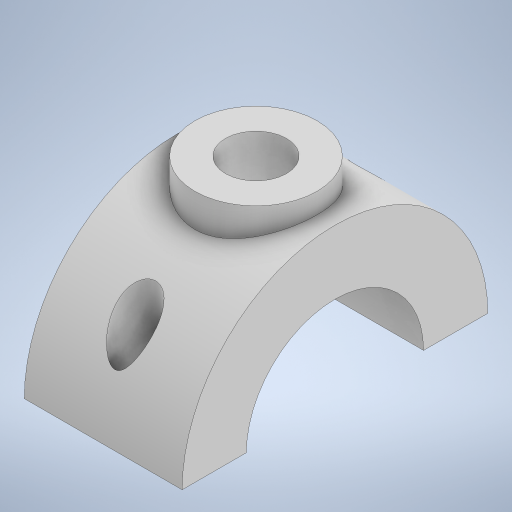
# Autodesk Inventor part: Parte1
Saved by Autodesk Inventor 2023 (Build 270158000, 158)
## iProperties
Created: 2022-11-03
Part Number: Parte1
Material: Generic
Document SubType Name: Modeling
Designer: ivanm
Density: 1 g/cm^3
Appearance: Default
Author: ivanm
Autodesk Inventor part; units mm, degrees
ref_plane "YZ Plane" through (0, 0, 0) normal (1, 0, 0) x (0, 1, 0)
ref_plane "XZ Plane" through (0, 0, 0) normal (0, 1, 0) x (-1, 0, 0)
ref_plane "XY Plane" through (0, 0, 0) normal (0, 0, 1) x (1, 0, 0)
sketch "Sketch1" plane through (0, 0, 0) normal (1, 0, 0) x (0, 1, 0)
  arc A0 (0, -8.7) -> (0, 8.7) centre (0, 0) ccw
  arc A1 (0, -15) -> (0, 15) centre (0, 0) ccw
  line L0 (0, 15) -> (0, 8.7)
  line L1 (0, -8.7) -> (0, -15)
  dimension "d0" = 17.4
  dimension "d1" = 30
  dimension "d17" = 6.3
  dimension "d18" = 6.3
  constraints: 4 end point, 4 point on circle, 3 coincident, 2 centre point, 2 vertical
  measures "d0" diameter of A0
  measures "d1" diameter of A1
  measures "d17" distance of L0.start L0.end
  measures "d18" distance of L1.start L1.end
extrude "Extrusion1" add sketch "Sketch1" along normal blind 15.5
ref_plane "Work Plane1" through (0, 15, 0) normal (0, -1, 0) x (1, 0, 0)
sketch "Sketch2" plane through (0, 15, 0) normal (0, -1, 0) x (1, 0, 0)
  line L0 (0, -15) -> (0, 15) projected
  line L1 (0, 15) -> (15.5, 15) projected
  line L2 (15.5, -15) -> (15.5, 15) projected
  line L3 (0, -15) -> (15.5, -15) projected
  line L4 (0, 0) -> (15.5, 0) construction
  line L5 (7.75, -15) -> (7.75, 15) construction
  circle A0 centre (7.75, 0) radius 6
  circle A1 centre (7.75, 0) radius 3
  dimension "d6" = 6
  dimension "d7" = 12
  constraints: 4 end point, 4 midpoint, 2 centre point, 1 coincident, 1 perpendicular
  measures "d6" diameter of A1
  measures "d7" diameter of A0
extrude "Extrusion2" add sketch "Sketch2" along normal up to surface contours A0 round surface about axis through (0, 0, 0) along (1, 0, 0) radius 15 far side no
extrude "Extrusion3" add sketch "Sketch2" against normal blind 2 contours A0
extrude "Extrusion4" cut sketch "Sketch2" along normal through all contours A1
ref_plane "Work Plane2" through (0, -8.7, 0) normal (0, -1, 0) x (1, 0, 0)
sketch "Sketch3" plane through (0, -8.7, 0) normal (0, -1, 0) x (1, 0, 0)
  spline S0 degree 5 poles (10.75, 0) (10.75, 0.1919) (10.7347, 0.3834) (10.7041, 0.5715) (10.6595, 0.7536) (10.4842, 1.2932) (10.3128, 1.6211) (10.104, 1.9046) (9.8731, 2.1435) (9.2912, 2.6088) (8.9274, 2.8036) (8.5449, 2.9327) (8.1539, 2.9984) (7.3698, 3.0016) (6.9775, 2.9389) (6.5935, 2.8124) (6.2279, 2.62) (5.7133, 2.2146) (5.5421, 2.0519) (5.3825, 1.8674) (5.238, 1.6607) (5.0376, 1.2915) (4.969, 1.1429) (4.9094, 0.9866) (4.86, 0.8234) (4.7677, 0.4105) (4.7372, 0.1545) (4.7351, -0.1058) (4.7615, -0.3627) (4.8805, -0.9375) (4.9927, -1.2467) (5.1399, -1.5242) (5.3101, -1.7688) (5.6294, -2.1312) (5.7684, -2.2647) (5.9146, -2.3841) (6.0665, -2.4898) (6.5084, -2.751) (6.8094, -2.8759) (7.1199, -2.9586) (7.4347, -3) (8.1471, -3) (8.5437, -2.9342) (8.9317, -2.8031) (9.3003, -2.6045) (9.8094, -2.1928) (9.9736, -2.0335) (10.127, -1.8538) (10.2662, -1.653) (10.5189, -1.1875) (10.6303, -0.9149) (10.7095, -0.6203) (10.75, -0.3119) (10.75, 0) knots 0 0 0 0 0 0 0.042105 0.042105 0.042105 0.042105 0.130974 0.130974 0.130974 0.130974 0.2493 0.2493 0.2493 0.2493 0.367924 0.367924 0.367924 0.367924 0.431887 0.431887 0.431887 0.431887 0.470966 0.470966 0.470966 0.470966 0.527372 0.527372 0.527372 0.527372 0.602951 0.602951 0.602951 0.602951 0.65513 0.65513 0.65513 0.65513 0.7503 0.7503 0.7503 0.7503 0.870161 0.870161 0.870161 0.870161 0.931934 0.931934 0.931934 0.931934 1 1 1 1 1 1 projected
  line L0 (0, 8.7) -> (0, -8.7) projected
  line L1 (0, -8.7) -> (15.5, -8.7) projected
  line L2 (15.5, 8.7) -> (15.5, -8.7) projected
  line L3 (0, 8.7) -> (15.5, 8.7) projected
  circle A0 centre (7.75, 0) radius 3 projected
  circle A1 centre (7.75, 0) radius 5
  point P0 (0, 0)
  dimension "d14" = 10
  constraints: 1 centre point, 1 coincident, 1 vertical alignment, 1 other
  measures "d14" diameter of A1
extrude "Extrusion5" cut sketch "Sketch3" against normal blind 20.4 contours A1
ref_plane "Work Plane3" through (0, -15, 0) normal (0, -1, 0) x (1, 0, 0)
sketch "Sketch4" plane through (0, -15, 0) normal (0, -1, 0) x (1, 0, 0)
  line L0 (0, 15) -> (0, 8.7) projected
  line L1 (0, 8.7) -> (15.5, 8.7) projected
  line L2 (15.5, 15) -> (15.5, 8.7) projected
  line L3 (0, 15) -> (15.5, 15) projected
  line L4 (0, -8.7) -> (0, -15) projected
  line L5 (0, -15) -> (15.5, -15) projected
  line L6 (15.5, -8.7) -> (15.5, -15) projected
  line L7 (0, -8.7) -> (15.5, -8.7) projected
  circle A0 centre (7.75, 11.85) radius 2
  circle A1 centre (7.75, -11.85) radius 2
  line L8 (15.5, 11.85) -> (0, 11.85) construction
  line L9 (7.75, 8.7) -> (7.75, 15) construction
  line L10 (7.75, -15) -> (7.75, -8.7) construction
  line L11 (15.5, -11.85) -> (0, -11.85) construction
  point P0 (0, 0)
  dimension "d19" = 4
  dimension "d20" = 4
  constraints: 10 midpoint, 8 end point, 2 centre point, 2 coincident
  measures "d19" diameter of A0
  measures "d20" diameter of A1
extrude "Extrusion6" cut sketch "Sketch4" against normal through all contours A0 | A1
equation "\"d18\" = d17"
equation "\"d20\" = d19"
body "Solid1"
